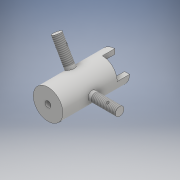
# Autodesk Inventor part: UntererRührerHalter
Saved by Autodesk Inventor 2017 (Build 210142000, 142)
## iProperties
Created: 2019-06-21
Part Number: UntererRührerHalter
Material: Generic
Document SubType Name: Modeling
Designer: Ole Simmering
Density: 1 g/cm^3
Appearance: Default
Author: Ole Simmering
Autodesk Inventor part; units mm, degrees
ref_plane "XZ Plane" through (0, 0, 0) normal (0, 1, 0) x (-1, 0, 0)
ref_plane "XY Plane" through (0, 0, 0) normal (0, 0, 1) x (1, 0, 0)
sketch "Sketch1" plane through (0, 0, 0) normal (0, 1, 0) x (-1, 0, 0)
  circle A0 centre (0, 0) radius 6
  dimension "d0" = 12
  constraints: 1 centre point, 1 coincident
  measures "d0" diameter of A0
extrude "Extrusion1" add sketch "Sketch1" along normal blind 2
sketch "Sketch2" plane through (0, 2, 0) normal (0, 1, 0) x (1, 0, 0)
  circle A0 centre (0, 0) radius 4
  circle A1 centre (0, 0) radius 6
  dimension "d3" = 8
  constraints: 2 centre point, 2 coincident
  measures "d3" diameter of A0
extrude "Extrusion2" add sketch "Sketch2" along normal blind 20
sketch "Sketch3" plane through (0, 22, 0) normal (0, 1, 0) x (1, 0, 0)
  arc A0 (-6, 0) -> (0, -6) centre (0, 0) ccw
  circle A1 centre (0, 0) radius 6 construction
  arc A2 (6, 0) -> (0, 6) centre (0, 0) ccw
  line L0 (0, -6) -> (0, -4)
  circle A3 centre (0, 0) radius 4 construction
  line L1 (0, 4) -> (0, 6)
  line L2 (6, 0) -> (4, 0)
  line L3 (-4, 0) -> (-6, 0)
  arc A4 (-4, 0) -> (0, -4) centre (0, 0) ccw
  arc A5 (4, 0) -> (0, 4) centre (0, 0) ccw
  constraints: 11 point on circle, 8 end point, 4 centre point, 4 coincident, 2 horizontal, 2 vertical, 1 vertical alignment, 1 other
extrude "Extrusion3" add sketch "Sketch3" along normal blind 5
ref_plane "Work Plane1" through (5, 0, 0) normal (1, 0, 0) x (0, 1, 0)
sketch "Sketch5" plane through (5, 0, 0) normal (1, 0, 0) x (0, 1, 0)
  line L0 (22, 0) -> (22, 6) construction
  line L1 (22, 6) -> (2, -6) construction
  line L2 (22, -6) -> (22, 0) construction
  line L3 (22, -6) -> (2, 6) construction
  circle A0 centre (12, 0) radius 1.75
  point P0 (0, 0)
  dimension "d10" = 3.5
  constraints: 4 end point, 1 centre point, 1 midpoint
  measures "d10" diameter of A0
extrude "Extrusion4" add sketch "Sketch5" along normal blind 12
pattern_circular "Circular Pattern1" count 3 over 360 about axis through (0, 0, 0) along (0, 1, 0) of "Extrusion4"
thread "Thread1" size "M3.5x0.6" class "6g" standard "ANSI Metric M Profile" length 10
thread "Thread2" size "M3.5x0.6" class "6g" standard "ANSI Metric M Profile" length 10
thread "Thread3" size "M3.5x0.6" class "6g" standard "ANSI Metric M Profile" length 10
ref_plane "Work Plane3" through (13, 12, 0) normal (1, 0, 0) x (0, 0, -1)
sketch "Sketch7" plane through (13, 12, 0) normal (1, 0, 0) x (0, 0, -1)
  circle A0 centre (0, 0) radius 1.75 construction
  arc A1 (0, 6.6281) -> (-5.7401, -3.3141) centre (0, 0) ccw construction
  line L0 (0, 0) -> (-5.7401, -3.3141) construction
  line L1 (0, 0) -> (0, 6.6281) construction
  point P0 (0, -12)
  dimension "d23" = 120
  constraints: 4 end point, 2 centre point, 2 point on circle, 1 coincident
  measures "d23" angle of L1 L0
sketch "Sketch8" plane through (0, 0, 0) normal (0, -1, 0) x (1, 0, 0)
  point P0 (0, 0)
  point P1 (0, 0)
  constraints: 1 coincident
hole "Hole1" at (0, 0, 0) direction (0, 1, 0) diameter 2.4 end through all
ref_plane "Work Plane5" through (13, 11, 1.7321) normal (0, -0.5, 0.8660254) x (1, 0, 0)
ref_plane "Work Plane4" through (13, 12, 0) normal (0, -0.5, 0.8660254) x (1, 0, 0)
sketch "Sketch10" plane through (13, 11, 1.7321) normal (0, -0.5, 0.8660254) x (1, 0, 0)
  line L0 (-7, -10.3923) -> (-7, 12.9904) construction
  line L1 (-7, 1.7737) -> (-7, -1.9186) construction
  point P0 (-13, -10.3923)
  point P1 (0, 0)
  dimension "d33" = 7
  constraints: 2 end point, 2 point on line
  measures "d33" distance from line of point (0, 0) L0
hole "Hole2" at (13, 11, 1.7321) direction (0, 0.5, -0.8660254) diameter 1 end through all
pattern_circular "Circular Pattern2" count 3 over 360 about axis through (0, 0, 0) along (0, 1, 0) of "Hole2"
body "Solid1"
